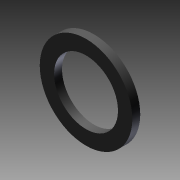
# Autodesk Inventor part: AT401P(WT)
Saved by Autodesk Inventor 2011 SP1 (Build 150282100, 282)
## iProperties
Created: 2013-12-24
Part Number: AT401P(WT)
Catalog Web Link: www.cadenas.de
Description: AT401P-O-ring, Natural rubber
Vendor: NKKSWITCHES
Document SubType Name: Modeling
Designer: PARTuser1
Manufacturer: NKKSWITCHES
Density: 1 g/cm^3
Category: PARTsolutions
Company: NKKSWITCHES
Title: AT401P
Author: Cadenas PARTsolutions
Comments: O-ring, Natural rubber
PSOL_IDENT_0: {$CADENAS_DATA\23d-libs\nkkswitches\toggle\wt\wt_accessories\at401p.prj},158 {VTYP=3D},{NB=AT401P(WT
PSOL_IDENT_1: )},{LINA=AT401P},{NN=AT401P},{DATE=26.06.2008 06:57:04},{GEOMDATE=26.06.2008 00:00:00},{VERSION=},{L
PSOL_IDENT_2: INEID=10},{LINESUBID=-1},{WBVAR=}  {NB=AT401P(WT)},{LINA=AT401P},{KT=DUMMY},{PN=AT401P},{D=0.689},{D
PSOL_IDENT_3: D=0.476},{T=0.059}
CNS_NN: AT401P
CNS_NT: O-ring, Natural rubber
CNS_NB: AT401P(WT)
CNS_NBSYN: $PN.(WT)
CNS_LINA: AT401P
CNS_PN: AT401P
CNS_D: 0.689
CNS_DD: 0.476
CNS_T: 0.059
SUPPLIER: NKKSWITCHES
ARTICLENO: AT401P(WT)
BOMINFO: AT401P
CREATOR: CADENAS GmbH
Autodesk Inventor part; units mm, degrees
sketch "Sketch_1" plane through (0, 0, 0) normal (0, 1, 0) x (-1, 0, 0)
  line L0 (0, 0.7493) -> (0, -0.7493)
  line L1 (-6.0452, 0.7493) -> (-8.7503, 0.7493)
  line L2 (-8.7503, 0.7493) -> (-8.7503, -0.7493)
  line L3 (-8.7503, -0.7493) -> (-6.0452, -0.7493)
  line L4 (-6.0452, -0.7493) -> (-6.0452, 0.7493)
  constraints: 10 end point
revolve "Revolution1" add sketch "Sketch_1" angle 360 about axis through (0, 0, 0.7493) along (0, 0, 1)
ref_plane "o_ring_XY" through (0, 0, 0.7493) normal (0, 0, 1) x (1, 0, 0)
ref_plane "o_ring_YZ" through (0, 0, 0.7493) normal (1, 0, 0) x (0, 1, 0)
ref_plane "o_ring_ZX" through (0, 0, 0.7493) normal (0, 1, 0) x (0, 0, 1)
ref_plane "o_ring_new_XY" through (0, 0, -0.7493) normal (0, 0, 1) x (1, 0, 0)
ref_plane "o_ring_new_YZ" through (0, 0, -0.7493) normal (1, 0, 0) x (0, 1, 0)
ref_plane "o_ring_new_ZX" through (0, 0, -0.7493) normal (0, 1, 0) x (0, 0, 1)
body "Solid1"
